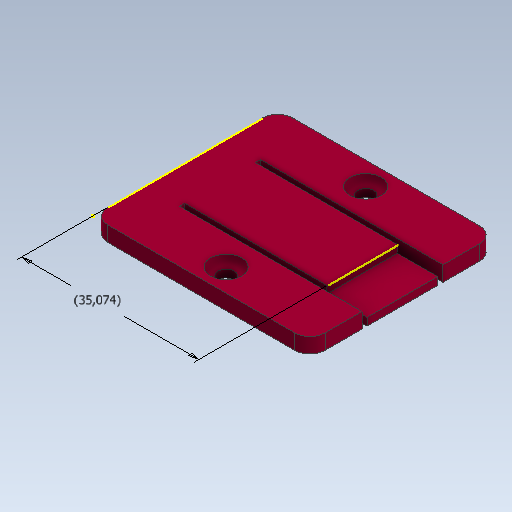
# Autodesk Inventor part: shelki
Saved by Autodesk Inventor 2020 (Build 240168000, 168)
## iProperties
Created: 2022-07-20
Part Number: shelki
Material: Типовые
Document SubType Name: Modeling
Designer: akapu
Density: 1 g/cm^3
Appearance: По умолчанию
Author: akapu
Autodesk Inventor part; units mm, degrees
ref_plane "YZ Plane" through (0, 0, 0) normal (1, 0, 0) x (0, 1, 0)
ref_plane "XZ Plane" through (0, 0, 0) normal (0, 1, 0) x (-1, 0, 0)
ref_plane "XY Plane" through (0, 0, 0) normal (0, 0, 1) x (1, 0, 0)
sketch "Эскиз1" plane through (0, 0, 0) normal (0, 1, 0) x (-1, 0, 0)
  line L0 (-3, 0) -> (-39.988, 0)
  line L1 (-42.988, -3) -> (-42.988, -33.6)
  line L2 (-39.988, -36.6) -> (-3, -36.6)
  line L3 (0, -33.6) -> (0, -3)
  arc A0 (-39.988, 0) -> (-42.988, -3) centre (-39.988, -3) ccw
  arc A1 (-42.988, -33.6) -> (-39.988, -36.6) centre (-39.988, -33.6) ccw
  arc A2 (-3, -36.6) -> (0, -33.6) centre (-3, -33.6) ccw
  arc A3 (0, -3) -> (-3, 0) centre (-3, -3) ccw
  line L4 (-42.988, 0) -> (-21.911, 0)
  line L5 (-21.911, 0) -> (-21.911, -4.5)
  line L6 (-21.911, -36.6) -> (-21.911, -32.1)
  circle A4 centre (-21.911, -4.5) radius 1.6
  circle A5 centre (-21.911, -32.1) radius 1.6
  line L7 (-21.911, -25.3) -> (-42.988, -25.3)
  line L8 (-21.911, -11.3) -> (-42.988, -11.3)
  line L9 (-21.911, -11.3) -> (-6.911, -11.3)
  line L10 (-6.911, -11.3) -> (-6.911, -25.3)
  line L11 (-6.911, -25.3) -> (-21.911, -25.3)
  line L12 (-6.911, -11.3) -> (-42.988, -11.3)
  line L13 (-42.988, -11.3) -> (-42.988, -10.3)
  line L14 (-42.988, -10.3) -> (-6.911, -10.3)
  line L15 (-6.911, -10.3) -> (-6.911, -11.3)
  line L16 (-6.911, -25.3) -> (-42.988, -25.3)
  line L17 (-42.988, -25.3) -> (-42.988, -26.3)
  line L18 (-42.988, -26.3) -> (-6.911, -26.3)
  line L19 (-6.911, -26.3) -> (-6.911, -25.3)
  point P0 (0, 0)
  point P1 (-42.988, -36.6)
  point P2 (0, -36.6)
  dimension "d0" = 42.988
  dimension "d1" = 36.6
  dimension "d2" = 3
  dimension "d3" = 21.077
  dimension "d4" = 4.5
  dimension "d5" = 4.5
  dimension "d6" = 3.2
  dimension "d7" = 3.2
  dimension "d11" = 1
  dimension "d12" = 1
  constraints: 40 end point, 14 point on line, 8 perpendicular, 8 point on circle, 8 tangent, 7 parallel, 6 centre point, 4 horizontal, 3 equal radius, 2 coincident
  measures "d0" distance of point (0, -36.6) point (-42.988, -36.6)
  measures "d1" distance of point (-42.988, -36.6) L4.start
  measures "d2" radius of A0
  measures "d3" distance of L4.start L4.end
  measures "d4" distance of L4.end L5.end
  measures "d5" distance of L6.start L6.end
  measures "d6" diameter of A4
  measures "d7" diameter of A5
  measures "d11" distance of L12.end L13.end
  measures "d12" distance of L17.end L16.end
extrude "Выдавливание1" add sketch "Эскиз1" along normal blind 3 contours A3 L3 A2 L2 A1 L1 L18 L19 L10 L15 L14 A0 L0
sketch "Эскиз4" plane through (6.911, 0, -26.3) normal (0, 0, 1) x (1, 0, 0)
  line L0 (36.077, 0) -> (36.077, 3) projected
  line L1 (36.077, 0) -> (26.077, 0)
  line L2 (36.077, 0) -> (33.077, 0) projected
  line L3 (36.077, 0) -> (36.077, 1.5)
  line L4 (36.077, 1.5) -> (28.077, 1.5)
  line L5 (36.077, 3) -> (0, 3) projected
  line L6 (0, 0) -> (0, 3) projected
  line L7 (0, 1.5) -> (26.077, 0)
  line L8 (28.077, 1.5) -> (28.1633, 3)
  line L9 (0, 3) -> (28.1633, 3)
  line L10 (0, 3) -> (36.077, 3) projected
  dimension "d18" = 10
  constraints: 12 end point, 2 collinear, 2 midpoint, 1 perpendicular, 1 point on line
  measures "d18" distance of L0.start L1.end
extrude "Выдавливание2" add sketch "Эскиз4" along normal blind 15 contours L1 L7 L6 L5 L8 L4 L0
sketch "Эскиз5" plane through (0, 3, 0) normal (0, 1, 0) x (1, 0, 0)
  line L0 (6.911, 11.3) -> (32.988, 11.3) projected
  line L1 (6.911, 10.3) -> (6.911, 26.3) projected
  line L2 (6.911, 11.3) -> (6.911, 26.3)
  line L3 (6.911, 26.3) -> (42.988, 26.3)
  line L4 (42.988, 33.6) -> (42.988, 11.3) projected
  line L5 (35.0743, 26.3) -> (42.988, 26.3) projected
  line L6 (42.988, 26.3) -> (42.988, 25.3)
  line L7 (42.988, 25.3) -> (6.911, 25.3)
  point P0 (0, 0)
  dimension "d22" = 1
  constraints: 8 end point, 2 perpendicular, 2 point on line, 1 collinear, 1 vertical
  measures "d22" distance of L3.end L6.end
extrude "Выдавливание3" cut sketch "Эскиз5" against normal blind 15
fillet "Сопряжение1" radius 1.5 2 edges at (23.511, 3, -4.5) (23.511, 3, -32.1) inverted yes
sketch "Эскиз6" plane through (0, 3, 0) normal (0, 1, 0) x (1, 0, 0)
  line L0 (0, 33.6) -> (0, 3) projected
  line L1 (35.0743, 25.3) -> (35.0743, 11.3) projected
  point P0 (0, 0)
  dimension "d26" = 35.0743
  measures "d26" distance between parallel lines of L0 L1
